Autodesk Inventor part; units mm, degrees
(part 2 of 2)
sketch "Sketch3" plane through (0, 0, 0) normal (0, 0, -1) x (-1, 0, 0)
  line L0 (0, 0) -> (-75.1754, 27.3616) construction
  line L1 (0, 0) -> (-66.0394, 45.153) construction
  line L2 (-75.1754, 27.3616) -> (-66.0394, 45.153) construction
  line L3 (0, 0) -> (-70, 0) construction
  arc A0 (-69.2544, 10.1895) -> (69.6176, 7.3067) centre (0, 0) ccw construction
  circle A1 centre (-75.1754, 27.3616) radius 4
  circle A2 centre (-66.0394, 45.153) radius 4
  circle A3 centre (1.6604, 79.9828) radius 17.5 construction
  circle A4 centre (0, 0) radius 17.5 construction
  arc A5 (61.3326, 86.2456) -> (-57.7006, 88.7167) centre (1.6604, 79.9828) ccw construction
  line L4 (-57.7006, 88.7167) -> (-69.2544, 10.1895) construction
  arc A6 (-69.2544, 10.1895) -> (69.6176, 7.3067) centre (0, 0) ccw construction
  line L5 (69.6176, 7.3067) -> (61.3326, 86.2456) construction
  line L6 (-62.4764, 16.2573) -> (-87.1754, 16.2573)
  line L7 (-87.1754, 16.2573) -> (-87.1754, 56.2573)
  line L8 (-87.1754, 56.2573) -> (-62.4764, 56.2573)
  line L9 (-62.4764, 56.2573) -> (-62.4764, 16.2573)
  line L10 (-62.4764, 16.2573) -> (-87.1754, 56.2573) construction
  line L11 (-87.1754, 16.2573) -> (-62.4764, 56.2573) construction
  point P0 (-74.8259, 36.2573)
  point P1 (-74.8259, 36.2573)
  point P2 (-70.6074, 36.2573)
  dimension "d8" = 80
  dimension "d9" = 20
  dimension "d10" = 20
  dimension "d11" = 8
  dimension "d12" = 40
  dimension "d13" = 12
  constraints: 20 end point, 4 midpoint, 2 centre point, 2 coincident, 2 horizontal, 2 parallel, 1 equal length, 1 equal radius, 1 horizontal alignment, 1 perpendicular, 1 point on circle, 1 point on line
  measures "d8" distance of L0.start L0.end
  measures "d9" distance of L0.end L1.end
  measures "d10" angle of L0 L3
  measures "d11" diameter of A1
  measures "d12" distance of L6.end L7.end
  measures "d13" distance from line of L0.end L7
extrude "Extrusion3" add sketch "Sketch3" against normal up to surface (12 mm away) contours A2 L9 L6 L7 L8
sketch "Sketch5" plane through (0, 0, 12) normal (0, 0, 1) x (1, 0, 0)
  circle A0 centre (-1.6604, 79.9828) radius 6.75 construction
  line L0 (-1.6604, 79.9828) -> (-1.6604, 14.9828) construction
  line L1 (87.1754, 56.2573) -> (87.1754, 16.2573) construction
  line L2 (87.1754, 36.2573) -> (71.2219, 36.2573) construction
  line L3 (58.9994, 52.7076) -> (83.4444, 52.7076) construction
  line L4 (83.4444, 52.7076) -> (83.4444, 19.807) construction
  line L5 (83.4444, 19.807) -> (58.9994, 19.807) construction
  line L6 (58.9994, 19.807) -> (58.9994, 52.7076) construction
  line L7 (58.9994, 52.7076) -> (83.4444, 19.807) construction
  line L8 (83.4444, 52.7076) -> (58.9994, 19.807) construction
  line L9 (-24.1604, 24.9828) -> (20.8396, 24.9828) construction
  line L10 (20.8396, 24.9828) -> (20.8396, 4.9828) construction
  line L11 (20.8396, 4.9828) -> (-24.1604, 4.9828) construction
  line L12 (-24.1604, 4.9828) -> (-24.1604, 24.9828) construction
  line L13 (-24.1604, 24.9828) -> (20.8396, 4.9828) construction
  line L14 (20.8396, 24.9828) -> (-24.1604, 4.9828) construction
  circle A1 centre (20.8396, 4.9828) radius 1.25
  circle A2 centre (20.8396, 24.9828) radius 1.25
  circle A3 centre (-24.1604, 24.9828) radius 1.25
  circle A4 centre (-24.1604, 4.9828) radius 1.25
  circle A5 centre (0, 0) radius 17.5 construction
  point P0 (0, 0)
  dimension "d18" = 65
  dimension "d19" = 2.5
  dimension "d20" = 45
  dimension "d21" = 20
  constraints: 28 end point, 5 midpoint, 4 centre point, 4 coincident, 4 parallel, 3 equal radius, 3 horizontal, 2 perpendicular, 1 vertical
  measures "d18" distance of L0.start L0.end
  measures "d19" diameter of A1
  measures "d20" distance of L10.end L11.end
  measures "d21" distance of L9.end L10.end
extrude "Extrusion5" [suppressed]
sketch "Sketch6" plane through (0, 0, 0) normal (0, 0, -1) x (-1, 0, 0)
  arc A0 (-63.6393, 48.353) -> (-64.6627, 41.3974) centre (-66.0394, 45.153) ccw projected
  line L0 (-63.6393, 48.353) -> (-64.6627, 41.3974) projected
  line L1 (-64.6627, 41.3974) -> (-63.6393, 48.353) projected
  circle A1 centre (-66.0394, 45.153) radius 4
  point P0 (0, 0)
  constraints: 1 coincident, 3 other
extrude "Extrusion6" cut sketch "Sketch6" against normal through all contours A1 L0
sketch "Sketch7" plane through (0, 0, 0) normal (0, 0, -1) x (-1, 0, 0)
  circle A0 centre (1.6604, 79.9828) radius 17.5 construction
  circle A1 centre (0, 0) radius 17.5 construction
  circle A2 centre (-66.0394, 45.153) radius 4 construction
  circle A3 centre (-75.1754, 27.3616) radius 4 construction
  line L0 (-68.3616, 16.2573) -> (-69.2544, 10.1895) construction
  arc A4 (-69.2544, 10.1895) -> (69.6176, 7.3067) centre (0, 0) ccw construction
  line L1 (69.6176, 7.3067) -> (61.3326, 86.2456) construction
  arc A5 (61.3326, 86.2456) -> (-57.7006, 88.7167) centre (1.6604, 79.9828) ccw construction
  line L2 (-57.7006, 88.7167) -> (-62.4764, 56.2573) construction
  line L3 (-87.1754, 56.2573) -> (-62.4764, 56.2573) construction
  line L4 (-87.1754, 16.2573) -> (-87.1754, 56.2573) construction
  line L5 (-68.3616, 16.2573) -> (-87.1754, 16.2573) construction
  arc A6 (-69.2544, 10.1895) -> (69.6176, 7.3067) centre (0, 0) ccw projected
  circle A7 centre (-69.2544, 10.1895) radius 1.905
  circle A8 centre (-1.4528, -69.9849) radius 1.905
  circle A9 centre (69.6176, 7.3067) radius 1.905
  arc A10 (61.3326, 86.2456) -> (-57.7006, 88.7167) centre (1.6604, 79.9828) ccw projected
  circle A11 centre (-57.7006, 88.7167) radius 1.905
  circle A12 centre (2.9056, 139.9698) radius 1.905
  line L6 (61.3326, 86.2456) -> (69.6176, 7.3067) projected
  circle A13 centre (61.3326, 86.2456) radius 1.905
  circle A14 centre (-69.2544, 10.1895) radius 4
  circle A15 centre (-1.4528, -69.9849) radius 4
  circle A16 centre (69.6176, 7.3067) radius 4
  circle A17 centre (61.3326, 86.2456) radius 4
  circle A18 centre (2.9056, 139.9698) radius 4
  line L7 (-62.4764, 56.2573) -> (-57.7006, 88.7167) projected
  circle A19 centre (-57.7006, 88.7167) radius 4
  dimension "d26" = 3.81
  dimension "d27" = 8
  constraints: 12 centre point, 10 equal radius, 8 coincident, 4 point on circle
  measures "d26" diameter of A7
  measures "d27" diameter of A14
extrude "Extrusion7" add sketch "Sketch7" against normal up to surface (12 mm away) contours A15 A6 A8 | A6 A8 A15 | A16 L6 A9 A6 | A6 A9 L6 A16 | A13 L6 A17 A10 | A10 A17 L6 A13 | A18 A10 A12 | A10 A12 A18 | A19 L7 A11 A10 | A10 A11 L7 A19 | A14
extrude "Extrusion8" cut sketch "Sketch7" against normal through all contours A8 A6 | A6 A8 | A9 L6 A6 | A6 L6 A9 | A7 | L6 A13 A10 | A10 A13 L6 | A12 A10 | A10 A12 | A11 L7 A10 | A10 L7 A11
sketch "Sketch8" plane through (0, 0, 12) normal (0, 0, 1) x (1, 0, 0)
  circle A0 centre (-69.6176, 7.3067) radius 1.905 construction
  circle A1 centre (69.2544, 10.1895) radius 1.905 construction
  arc A2 (-6.8998, 139.7536) -> (-60.7827, 90.2077) centre (-1.6604, 79.9828) ccw construction
  arc A3 (-60.7827, 90.2077) -> (-61.7501, 82.2675) centre (-61.3326, 86.2456) ccw construction
  line L0 (-61.7501, 82.2675) -> (-69.2001, 11.2848) construction
  arc A4 (-69.2001, 11.2848) -> (-69.9213, 3.3182) centre (-69.6176, 7.3067) ccw construction
  arc A5 (-69.9213, 3.3182) -> (-2.5471, -69.9536) centre (0, 0) ccw construction
  arc A6 (-2.5471, -69.9536) -> (5.448, -69.7877) centre (1.4528, -69.9849) ccw construction
  arc A7 (5.448, -69.7877) -> (69.7234, 6.2171) centre (0, 0) ccw construction
  arc A8 (69.7234, 6.2171) -> (68.6721, 14.1469) centre (69.2544, 10.1895) ccw construction
  line L1 (68.6721, 14.1469) -> (68.3616, 16.2573) construction
  line L2 (87.1754, 16.2573) -> (68.3616, 16.2573) construction
  line L3 (87.1754, 56.2573) -> (87.1754, 16.2573) construction
  line L4 (62.4764, 56.2573) -> (87.1754, 56.2573) construction
  line L5 (62.4764, 56.2573) -> (58.2828, 84.7593) construction
  arc A9 (58.2828, 84.7593) -> (56.9867, 92.6524) centre (57.7006, 88.7167) ccw construction
  arc A10 (56.9867, 92.6524) -> (1.094, 139.9195) centre (-1.6604, 79.9828) ccw construction
  arc A11 (1.094, 139.9195) -> (-6.8998, 139.7536) centre (-2.9056, 139.9698) ccw construction
  circle A12 centre (57.7006, 88.7167) radius 1.905 construction
  circle A13 centre (-2.9056, 139.9698) radius 1.905 construction
  circle A14 centre (-61.3326, 86.2456) radius 1.905 construction
  circle A15 centre (1.4528, -69.9849) radius 1.905 construction
  circle A16 centre (75.1754, 27.3616) radius 4 construction
  circle A17 centre (66.0394, 45.153) radius 4 construction
  line L6 (87.1754, 36.2573) -> (69.1754, 36.2573) construction
  line L7 (55.1754, 19.7573) -> (83.1754, 19.7573) construction
  line L8 (83.1754, 19.7573) -> (83.1754, 52.7573) construction
  line L9 (83.1754, 52.7573) -> (55.1754, 52.7573) construction
  line L10 (55.1754, 52.7573) -> (55.1754, 19.7573) construction
  line L11 (55.1754, 19.7573) -> (83.1754, 52.7573) construction
  line L12 (83.1754, 19.7573) -> (55.1754, 52.7573) construction
  circle A18 centre (83.1754, 52.7573) radius 1.397
  circle A19 centre (83.1754, 19.7573) radius 1.397
  circle A20 centre (55.1754, 19.7573) radius 1.397
  circle A21 centre (55.1754, 52.7573) radius 1.397
  dimension "d32" = 2.794
  dimension "d33" = 4
  dimension "d34" = 33
  dimension "d35" = 28
  constraints: 14 end point, 4 centre point, 4 coincident, 3 equal radius, 3 midpoint, 2 horizontal, 2 parallel, 1 perpendicular
  measures "d32" diameter of A18
  measures "d33" distance between parallel lines of L3 L8
  measures "d34" distance of L7.end L8.end
  measures "d35" distance of L8.end L9.end
extrude "Extrusion9" cut sketch "Sketch8" against normal through all
sketch "Sketch9" plane through (0, 0, 0) normal (0, 0, -1) x (-1, 0, 0)
  circle A0 centre (-55.1754, 19.7573) radius 1.397 projected
  circle A1 centre (-83.1754, 52.7573) radius 1.397 projected
  circle A2 centre (-83.1754, 19.7573) radius 1.397 projected
  circle A3 centre (-55.1754, 52.7573) radius 1.397 projected
  circle A4 centre (2.9056, 139.9698) radius 1.905 projected
  circle A5 centre (-1.4528, -69.9849) radius 1.905 projected
  circle A6 centre (61.3326, 86.2456) radius 1.905 projected
  circle A7 centre (-57.7006, 88.7167) radius 1.905 projected
  arc A8 (6.8998, 139.7536) -> (-1.094, 139.9195) centre (2.9056, 139.9698) ccw projected
  arc A9 (-1.094, 139.9195) -> (-56.9867, 92.6524) centre (1.6604, 79.9828) ccw projected
  arc A10 (-56.9867, 92.6524) -> (-58.2828, 84.7593) centre (-57.7006, 88.7167) ccw projected
  line L0 (-58.2828, 84.7593) -> (-62.4764, 56.2573) projected
  line L1 (-87.1754, 56.2573) -> (-62.4764, 56.2573) projected
  line L2 (-87.1754, 16.2573) -> (-87.1754, 56.2573) projected
  line L3 (-68.3616, 16.2573) -> (-87.1754, 16.2573) projected
  line L4 (-68.3616, 16.2573) -> (-68.6721, 14.1469) projected
  arc A11 (-68.6721, 14.1469) -> (-69.7234, 6.2171) centre (-69.2544, 10.1895) ccw projected
  arc A12 (-69.7234, 6.2171) -> (-5.448, -69.7877) centre (0, 0) ccw projected
  arc A13 (-5.448, -69.7877) -> (2.5471, -69.9536) centre (-1.4528, -69.9849) ccw projected
  arc A14 (2.5471, -69.9536) -> (69.9213, 3.3182) centre (0, 0) ccw projected
  arc A15 (69.9213, 3.3182) -> (69.2001, 11.2848) centre (69.6176, 7.3067) ccw projected
  line L5 (69.2001, 11.2848) -> (61.7501, 82.2675) projected
  arc A16 (61.7501, 82.2675) -> (60.7827, 90.2077) centre (61.3326, 86.2456) ccw projected
  arc A17 (60.7827, 90.2077) -> (6.8998, 139.7536) centre (1.6604, 79.9828) ccw projected
  circle A18 centre (-69.2544, 10.1895) radius 1.905 projected
  circle A19 centre (69.6176, 7.3067) radius 1.905 projected
  circle A20 centre (1.6604, 79.9828) radius 17.5 projected
  circle A21 centre (0, 0) radius 17.5 projected
  circle A22 centre (-66.0394, 45.153) radius 4 projected
  circle A23 centre (-75.1754, 27.3616) radius 4 projected
  line L6 (-87.1754, 16.2573) -> (-72.4115, 7.7334)
  arc A24 (-68.6721, 14.1469) -> (-69.7234, 6.2171) centre (-69.2544, 10.1895) ccw projected
  dimension "d38" = 30
  constraints: 2 end point, 2 point on circle
  measures "d38" angle of L3 L6
ref_plane "Work Plane2" through (48.3454, 15.3651, 12) normal (0, 0, -1) x (0, 1, 0)
extrude "Extrusion10" add sketch "Sketch9" against normal up to surface (12 mm away) contours L3 L4 A11 L6
sketch "Sketch10" plane through (0, 0, 12) normal (0, 0, 1) x (1, 0, 0)
  line L0 (-130.7584, 64.7011) -> (20.7847, 170.8128)
  line L1 (20.7847, 170.8128) -> (134.3528, 8.6206)
  line L2 (134.3528, 8.6206) -> (-17.1903, -97.491)
  line L3 (-17.1903, -97.491) -> (-130.7584, 64.7011)
  arc A0 (-2.5471, -69.9536) -> (5.448, -69.7877) centre (1.4528, -69.9849) ccw projected
  arc A1 (-6.8998, 139.7536) -> (-60.7827, 90.2077) centre (-1.6604, 79.9828) ccw projected
  arc A2 (-69.9213, 3.3182) -> (-2.5471, -69.9536) centre (0, 0) ccw projected
  line L4 (87.1754, 56.2573) -> (87.1754, 16.2573) projected
  arc A3 (5.448, -69.7877) -> (69.7234, 6.2171) centre (0, 0) ccw projected
  dimension "d41" = 198
  dimension "d42" = 185
  dimension "d43" = 35
  constraints: 8 end point, 2 parallel, 2 tangent, 1 perpendicular
  measures "d41" distance of L2.end L0.start
  measures "d42" distance of L0.start L0.end
  measures "d43" angle of L1 L4
body "Solid1"
